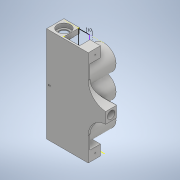
# Autodesk Inventor part: rearAxelHolder 10-29
Saved by Autodesk Inventor 2020 (Build 240168000, 168)
## iProperties
Created: 2019-10-24
Part Number: rearAxelHolder 10-29
Material: Generic
Document SubType Name: Modeling
Designer: Aditya Kendre
Density: 1 g/cm^3
Appearance: Default
Author: Aditya Kendre
## iProperties of the stored document rearAxelHolder 10-24_3DPrint.ipt
Created: 2019-10-24
Part Number: rearAxelHolder 10-24_3DPrint
Material: Generic
Document SubType Name: Modeling
Designer: Aditya Kendre
Density: 1 g/cm^3
Appearance: Default
Author: Aditya Kendre
Autodesk Inventor part; units mm, degrees
ref_plane "YZ Plane" through (0, 0, 0) normal (1, 0, 0) x (0, 1, 0)
ref_plane "XZ Plane" through (0, 0, 0) normal (0, 1, 0) x (-1, 0, 0)
ref_plane "XY Plane" through (0, 0, 0) normal (0, 0, 1) x (1, 0, 0)
sketch "Sketch1" plane through (0, 0, 0) normal (0, 1, 0) x (-1, 0, 0)
  line L0 (0, 0) -> (25, 0)
  line L1 (25, 0) -> (25, -165)
  line L2 (25, -165) -> (0, -165)
  line L3 (0, -165) -> (0, 0)
  dimension "d0" = 25
  dimension "d1" = 165
  constraints: 8 end point, 2 parallel, 1 horizontal, 1 perpendicular
  measures "d0" distance of L1.end L2.end
  measures "d1" distance of L0.end L1.end
extrude "Extrusion1" add sketch "Sketch1" along normal blind 3
sketch "Sketch2" plane through (0, 3, 0) normal (0, 1, 0) x (1, 0, 0)
  line L0 (0, 0) -> (0, 165) projected
  line L1 (-25, 165) -> (-25, 0) projected
  line L2 (0, 0) -> (-25, 0)
  line L3 (-25, 0) -> (-25, 8.5)
  line L4 (-25, 8.5) -> (0, 8.5)
  line L5 (0, 8.5) -> (0, 0)
  line L6 (-25, 165) -> (0, 165)
  line L7 (0, 165) -> (0, 156.5)
  line L8 (0, 156.5) -> (-25, 156.5)
  line L9 (-25, 156.5) -> (-25, 165)
  dimension "d4" = 8.5
  dimension "d5" = 8.5
  constraints: 16 end point, 4 parallel, 2 horizontal, 2 perpendicular, 2 point on line
  measures "d4" distance of L2.end L3.end
  measures "d5" distance of L6.end L7.end
extrude "Extrusion2" add sketch "Sketch2" along normal blind 25 contours L2 L1 L4 L0 | L8 L1 L6 L0
sketch "Sketch3" plane through (-25, 0, 0) normal (0, 0, 1) x (1, 0, 0)
  line L0 (0, 3) -> (0, 28) construction
  line L1 (25, 3) -> (25, 28) construction
  line L2 (0, 28) -> (25, 28) construction
  line L3 (25, 28) -> (25, 3) construction
  line L4 (25, 3) -> (0, 3) construction
  line L5 (0, 3) -> (0, 28) construction
  circle A0 centre (12.5, 15.5) radius 11.375
  point P0 (25, 0)
  dimension "d8" = 25
  dimension "d9" = 22.75
  constraints: 8 end point, 2 parallel, 1 centre point, 1 horizontal, 1 perpendicular
  measures "d8" distance of L2.end L1.start
  measures "d9" diameter of A0
extrude "Extrusion3" cut sketch "Sketch3" against normal blind 7.1
sketch "Sketch4" plane through (-25, 0, 0) normal (0, 0, 1) x (1, 0, 0)
  circle A0 centre (12.5, 15.5) radius 11.375 projected
  circle A1 centre (12.5, 15.5) radius 7.75
  point P0 (25, 0)
  dimension "d12" = 15.5
  constraints: 1 centre point, 1 coincident
  measures "d12" diameter of A1
extrude "Extrusion4" cut sketch "Sketch4" against normal blind 165 contours A1
sketch "Sketch5" plane through (0, 0, -165) normal (0, 0, -1) x (-1, 0, 0)
  circle A0 centre (12.5, 15.5) radius 7.75 projected
  circle A1 centre (12.5, 15.5) radius 11
  point P0 (0, 0)
  constraints: 1 centre point, 1 coincident
extrude "Extrusion5" cut sketch "Sketch5" against normal blind 7.1
sketch "Sketch6" plane through (0, 3, 0) normal (0, 1, 0) x (1, 0, 0)
  line L0 (-25, 156.5) -> (-25, 8.5) projected
  line L1 (-20.25, 8.5) -> (-4.75, 8.5) projected
  line L2 (-25, 156.5) -> (-20, 156.5)
  line L3 (-20, 156.5) -> (-20, 8.5)
  line L4 (-20, 8.5) -> (-25, 8.5)
  line L5 (-25, 8.5) -> (-25, 156.5)
  line L6 (0, 8.5) -> (0, 156.5) projected
  line L7 (-4.75, 156.5) -> (-20.25, 156.5) projected
  line L8 (0, 8.5) -> (-5, 8.5)
  line L9 (-5, 8.5) -> (-5, 156.5)
  line L10 (-5, 156.5) -> (0, 156.5)
  line L11 (0, 156.5) -> (0, 8.5)
  point P0 (0, 0)
  dimension "d17" = 5
  dimension "d18" = 5
  constraints: 16 end point, 4 parallel, 2 horizontal, 2 perpendicular, 2 point on line
  measures "d17" distance of L3.end L4.end
  measures "d18" distance of L9.end L10.end
extrude "Extrusion6" add sketch "Sketch6" along normal blind 10 contours L2 L3 L1 L4 L0 | L7 L10 L6 L8 L1 L9
fillet "Fillet1" radius 2 2 edges at (-5, 13, -82.5) (-20, 13, -82.5)
sketch "Sketch7" plane through (0, 0, 0) normal (1, 0, 0) x (0, 0, -1)
  line L0 (165, 0) -> (0, 0) projected
  line L1 (0, 0) -> (16, 0)
  line L2 (16, 0) -> (16, 8)
  line L3 (16, 8) -> (0, 8)
  line L4 (0, 8) -> (0, 0)
  line L5 (165, 0) -> (149, 0)
  line L6 (149, 0) -> (149, 8)
  line L7 (149, 8) -> (165, 8)
  line L8 (165, 8) -> (165, 0)
  line L9 (0, 28) -> (8.5, 28) projected
  line L10 (0, 28) -> (16, 28)
  line L11 (16, 28) -> (16, 20)
  line L12 (16, 20) -> (0, 20)
  line L13 (0, 20) -> (0, 28)
  line L14 (165, 0) -> (165, 28) projected
  line L15 (165, 28) -> (149, 28)
  line L16 (149, 28) -> (149, 20)
  line L17 (149, 20) -> (165, 20)
  line L18 (165, 20) -> (165, 28)
  dimension "d22" = 16
  dimension "d23" = 8
  dimension "d24" = 16
  dimension "d25" = 16
  dimension "d26" = 8
  constraints: 32 end point, 8 parallel, 4 horizontal, 4 perpendicular, 3 point on line
  measures "d22" distance of L3.end L2.end
  measures "d23" distance of L2.end L1.end
  measures "d24" distance of L6.end L7.end
  measures "d25" distance of L11.end L12.end
  measures "d26" distance of L10.end L11.end
extrude "Extrusion7" add sketch "Sketch7" along normal blind 45
fillet "Fillet2" radius 6 2 edges at (0, 24, -156.5) (0, 24, -8.5)
sketch "Sketch8" plane through (45, 0, 0) normal (1, 0, 0) x (0, 0, -1)
  line L0 (8.5, 20) -> (0, 20) construction
  line L1 (16, 28) -> (16, 20) construction
  line L2 (0, 20) -> (16, 28) construction
  line L3 (0, 0) -> (165, 0) construction
  line L4 (16, 8) -> (16, 0) construction
  line L5 (0, 0) -> (16, 8) construction
  line L6 (150.5, 28) -> (149, 28) construction
  line L7 (165, 8) -> (165, 20) construction
  line L8 (149, 28) -> (165, 20) construction
  line L9 (149, 0) -> (149, 8) construction
  line L10 (149, 8) -> (165, 0) construction
  line L11 (163.125, 22.25) -> (150.875, 22.25)
  line L12 (150.875, 22.25) -> (150.875, 25.75)
  line L13 (150.875, 25.75) -> (163.125, 25.75)
  line L14 (163.125, 25.75) -> (163.125, 22.25)
  line L15 (163.125, 22.25) -> (150.875, 25.75) construction
  line L16 (150.875, 22.25) -> (163.125, 25.75) construction
  line L17 (163.125, 2.25) -> (150.875, 2.25)
  line L18 (150.875, 2.25) -> (150.875, 5.75)
  line L19 (150.875, 5.75) -> (163.125, 5.75)
  line L20 (163.125, 5.75) -> (163.125, 2.25)
  line L21 (163.125, 2.25) -> (150.875, 5.75) construction
  line L22 (150.875, 2.25) -> (163.125, 5.75) construction
  line L23 (14.125, 22.25) -> (1.875, 22.25)
  line L24 (1.875, 22.25) -> (1.875, 25.75)
  line L25 (1.875, 25.75) -> (14.125, 25.75)
  line L26 (14.125, 25.75) -> (14.125, 22.25)
  line L27 (14.125, 22.25) -> (1.875, 25.75) construction
  line L28 (1.875, 22.25) -> (14.125, 25.75) construction
  line L29 (14.125, 2.25) -> (1.875, 2.25)
  line L30 (1.875, 2.25) -> (1.875, 5.75)
  line L31 (1.875, 5.75) -> (14.125, 5.75)
  line L32 (14.125, 5.75) -> (14.125, 2.25)
  line L33 (14.125, 2.25) -> (1.875, 5.75) construction
  line L34 (1.875, 2.25) -> (14.125, 5.75) construction
  point P0 (157, 24)
  point P1 (157, 4)
  point P2 (8, 24)
  point P3 (8, 4)
  dimension "d30" = 12.25
  dimension "d31" = 3.5
  dimension "d32" = 12.25
  dimension "d33" = 3.5
  dimension "d34" = 12.25
  dimension "d35" = 12.25
  dimension "d36" = 3.5
  constraints: 56 end point, 12 midpoint, 8 parallel, 4 horizontal, 4 perpendicular, 1 point on line
  measures "d30" distance of L12.end L13.end
  measures "d31" distance of L11.end L12.end
  measures "d32" distance of L18.end L19.end
  measures "d33" distance of L17.end L18.end
  measures "d34" distance of L24.end L25.end
  measures "d35" distance of L30.end L31.end
  measures "d36" distance of L29.end L30.end
extrude "Extrusion8" cut sketch "Sketch8" against normal blind 40
sketch "Sketch9" plane through (0, 8, 0) normal (0, 1, 0) x (1, 0, 0)
  line L0 (0, 0) -> (0, 16) construction
  line L1 (0, 8) -> (0, 9) construction
  line L2 (45, 1.875) -> (45, 14.125) construction
  line L3 (0, 9) -> (45, 9) construction
  line L4 (45, 9) -> (45, 7) construction
  line L5 (45, 7) -> (0, 7) construction
  line L6 (0, 7) -> (0, 9) construction
  line L7 (0, 9) -> (45, 9)
  line L8 (45, 9) -> (45, 7)
  line L9 (45, 7) -> (0, 7)
  line L10 (0, 7) -> (0, 9)
  line L11 (0, 149) -> (0, 165) construction
  line L12 (0, 149) -> (0, 157) construction
  line L13 (0, 157) -> (0, 158) construction
  line L14 (45, 165) -> (45, 149) projected
  line L15 (0, 158) -> (45, 158)
  line L16 (45, 158) -> (45, 156)
  line L17 (45, 156) -> (0, 156)
  line L18 (0, 156) -> (0, 158)
  dimension "d39" = 1
  dimension "d40" = 2
  dimension "d41" = 8
  dimension "d42" = 1
  dimension "d43" = 2
  constraints: 30 end point, 6 parallel, 4 point on line, 3 horizontal, 3 perpendicular, 1 midpoint, 1 vertical
  measures "d39" distance of L1.start L1.end
  measures "d40" distance of L3.end L4.end
  measures "d41" distance of L11.start L12.end
  measures "d42" distance of L12.end L13.end
  measures "d43" distance of L15.end L16.end
extrude "Extrusion9" add sketch "Sketch9" along normal blind 12
fillet "Fillet3" radius 6 2 edges at (0, 16.5, -156.5) (0, 16.5, -8.5)
sketch "Sketch10" plane through (-25, 0, -165) normal (0, 0, -1) x (-1, 0, 0)
  circle A0 centre (-12.5, 15.5) radius 11.375 projected
  circle A1 centre (-12.5, 15.5) radius 11.375
  point P0 (-25, 0)
  constraints: 1 centre point, 1 coincident
extrude "Extrusion10" cut sketch "Sketch10" against normal blind 7.1
sketch "Sketch11" plane through (0, 0, 0) normal (0, -1, 0) x (1, 0, 0)
  line L0 (0, -16) -> (45, -16) projected
  line L1 (0, -149) -> (0, -16) projected
  line L2 (45, -16) -> (0, -16)
  line L3 (0, -16) -> (0, -149)
  line L4 (0, -149) -> (45, -149)
  line L5 (45, -149) -> (45, -16)
  point P0 (0, 0)
  constraints: 8 end point, 2 parallel, 1 horizontal, 1 perpendicular
extrude "Extrusion11" add sketch "Sketch11" against normal blind 3
sketch "Sketch12" plane through (0, 3, 0) normal (0, 1, 0) x (1, 0, 0)
  point P0 (0, 0)
sketch "Sketch13" plane through (0, 3, 0) normal (0, 1, 0) x (1, 0, 0)
  point P0 (0, 0)
sketch "Sketch14" plane through (0, 3, 0) normal (0, 1, 0) x (1, 0, 0)
  line L0 (45, 16) -> (45, 0) construction
  line L1 (0, 149) -> (45, 149) construction
  line L2 (45, 16) -> (3, 16) construction
  line L3 (3, 16) -> (3, 149) construction
  line L4 (3, 149) -> (45, 149) construction
  line L5 (45, 149) -> (45, 16) construction
  line L6 (3, 16) -> (45, 149) construction
  circle A0 centre (24, 82.5) radius 21
  circle A1 centre (24, 82.5) radius 19.375
  line L7 (24, 82.5) -> (24, 124.5) construction
  circle A2 centre (24, 124.5) radius 21
  circle A3 centre (24, 124.5) radius 19.375
  line L8 (24, 82.5) -> (24, 40.5) construction
  circle A4 centre (24, 40.5) radius 21
  circle A5 centre (24, 40.5) radius 19.375
  point P0 (0, 0)
  dimension "d51" = 42
  dimension "d52" = 38.75
  dimension "d53" = 42
  dimension "d54" = 38.75
  dimension "d55" = 42
  dimension "d56" = 38.75
  constraints: 14 end point, 6 centre point, 5 coincident, 2 parallel, 2 tangent, 2 vertical, 1 horizontal, 1 midpoint, 1 perpendicular, 1 point on line
  measures "d51" distance of L3.end L4.end
  measures "d52" diameter of A1
  measures "d53" distance of L7.start L7.end
  measures "d54" diameter of A3
  measures "d55" distance of L7.start L8.end
  measures "d56" diameter of A5
extrude "Extrusion12" add sketch "Sketch14" along normal blind 45
sketch "Sketch15" plane through (24, 48, -40.5) normal (0, 1, 0) x (1, 0, 0)
  line L0 (0, 20.1158) -> (-2, 20.1158)
  line L1 (-2, 20.1158) -> (-2, 21.9714)
  line L2 (-2, 21.9714) -> (0, 21.9714)
  line L3 (0, 21.9714) -> (0, 20.1158)
  line L4 (-2, 21.9714) -> (2, 21.9714)
  line L5 (2, 21.9714) -> (2, 20.1158)
  line L6 (2, 20.1158) -> (-2, 20.1158)
  line L7 (-2, 20.1158) -> (-2, 21.9714)
  line L8 (0, 62.262) -> (-2, 62.262)
  line L9 (-2, 62.262) -> (-2, 63.8269)
  line L10 (-2, 63.8269) -> (0, 63.8269)
  line L11 (0, 63.8269) -> (0, 62.262)
  line L12 (-2, 63.8269) -> (2, 63.8269)
  line L13 (2, 63.8269) -> (2, 62.262)
  line L14 (2, 62.262) -> (-2, 62.262)
  line L15 (-2, 62.262) -> (-2, 63.8269)
  point P0 (-24, -40.5)
  dimension "d59" = 2
  dimension "d60" = 4
  dimension "d61" = 2
  dimension "d62" = 4
  constraints: 32 end point, 8 parallel, 4 horizontal, 4 perpendicular, 3 point on line
  measures "d59" distance of L1.end L2.end
  measures "d60" distance of L5.end L6.end
  measures "d61" distance of L9.end L10.end
  measures "d62" distance of L13.end L14.end
extrude "Extrusion13" add sketch "Sketch15" against normal blind 45
sketch "Sketch16" plane through (0, 28, 0) normal (0, 1, 0) x (1, 0, 0)
  circle A0 centre (24, 40.5) radius 19.375 construction
  line L0 (24, 40.5) -> (24, 0) construction
  line L1 (24, 0) -> (14, 0) construction
  line L2 (-25, 0) -> (45, 0) construction
  line L3 (0, 165) -> (45, 165) projected
  line L4 (19, 0) -> (0, 0)
  line L5 (0, 0) -> (0, 165)
  line L6 (0, 165) -> (19, 165)
  line L7 (19, 165) -> (19, 0)
  dimension "d65" = 10
  constraints: 12 end point, 2 parallel, 2 point on line, 1 horizontal, 1 perpendicular, 1 vertical
  measures "d65" distance of L0.end L1.end
sketch "Sketch17" plane through (0, 8, 0) normal (0, 1, 0) x (1, 0, 0)
  line L0 (0, 14.5) -> (0, 16) projected
  line L1 (-25, 0) -> (45, 0) projected
  line L2 (0, 16) -> (45, 16)
  line L3 (45, 16) -> (45, 0)
  line L4 (45, 0) -> (0, 0)
  line L5 (0, 0) -> (0, 16)
  line L6 (0, 165) -> (45, 165) projected
  line L7 (0, 149) -> (45, 149) projected
  line L8 (0, 165) -> (45, 165)
  line L9 (45, 165) -> (45, 149)
  line L10 (45, 149) -> (0, 149)
  line L11 (0, 149) -> (0, 165)
  constraints: 16 end point, 4 parallel, 2 horizontal, 2 perpendicular
extrude "Extrusion14" add sketch "Sketch17" along normal blind 12
sketch "Sketch18" plane through (-25, 0, -165) normal (-1, 0, 0) x (0, 0, 1)
  line L0 (0, 28) -> (16, 28) projected
  line L1 (156.5, 13) -> (8.5, 13) projected
  line L2 (0, 28) -> (8.5, 28)
  line L3 (8.5, 28) -> (8.5, 13)
  line L4 (8.5, 13) -> (0, 13)
  line L5 (0, 13) -> (0, 28)
  line L6 (156.5, 13) -> (156.5, 28) projected
  line L7 (165, 26.875) -> (165, 4.125) projected
  line L8 (156.5, 28) -> (165, 28)
  line L9 (165, 28) -> (165, 13)
  line L10 (165, 13) -> (156.5, 13)
  line L11 (156.5, 13) -> (156.5, 28)
  line L12 (165, 0) -> (0, 0)
  line L13 (0, 0) -> (0, 13)
  line L14 (0, 13) -> (165, 13)
  line L15 (165, 13) -> (165, 0)
  constraints: 24 end point, 6 parallel, 3 horizontal, 3 perpendicular, 2 point on line
extrude "Extrusion15" add sketch "Sketch18" along normal blind 2
sketch "Sketch19" plane through (0, 28, 0) normal (0, 1, 0) x (1, 0, 0)
  line L0 (45, 16) -> (45, 0) projected
  line L1 (0, 16) -> (0, 149) projected
  line L2 (45, 0) -> (0, 0)
  line L3 (0, 0) -> (0, 16)
  line L4 (0, 16) -> (45, 16)
  line L5 (45, 16) -> (45, 0)
  line L6 (-22, 8.5) -> (-27, 8.5) projected
  line L7 (0, 0) -> (-27, 0)
  line L8 (-27, 0) -> (-27, 8.5)
  line L9 (-27, 8.5) -> (0, 8.5)
  line L10 (0, 8.5) -> (0, 0)
  line L11 (0, 149) -> (45, 149) projected
  line L12 (-27, 165) -> (45, 165) projected
  line L13 (45, 149) -> (0, 149)
  line L14 (0, 149) -> (0, 165)
  line L15 (0, 165) -> (45, 165)
  line L16 (45, 165) -> (45, 149)
  line L17 (-27, 156.5) -> (-22, 156.5) projected
  line L18 (-27, 156.5) -> (0, 156.5)
  line L19 (0, 156.5) -> (0, 165)
  line L20 (0, 165) -> (-27, 165)
  line L21 (-27, 165) -> (-27, 156.5)
  arc A0 (0, 150.5) -> (-6, 156.5) centre (-6, 150.5) ccw projected
  arc A1 (0, 150.5) -> (-6, 156.5) centre (-6, 150.5) ccw
  arc A2 (-6, 8.5) -> (0, 14.5) centre (-6, 14.5) ccw projected
  arc A3 (-6, 8.5) -> (0, 14.5) centre (-6, 14.5) ccw
  constraints: 32 end point, 8 parallel, 5 point on circle, 4 horizontal, 4 perpendicular, 3 point on line, 2 centre point
extrude "Extrusion16" add sketch "Sketch19" along normal blind 2
sketch "Sketch20" plane through (-27, 0, -165) normal (-1, 0, 0) x (0, 0, 1)
  line L0 (83.5, 4) -> (81.5, 4)
  line L1 (81.5, 4) -> (81.5, 6)
  line L2 (81.5, 6) -> (83.5, 6)
  line L3 (83.5, 6) -> (83.5, 4)
  line L4 (83.5, 4) -> (81.5, 6) construction
  line L5 (81.5, 4) -> (83.5, 6) construction
  point P0 (165, 0)
  point P1 (82.5, 5000)
  point P2 (82.5, 5)
  dimension "d72" = 2
  dimension "d73" = 2
  constraints: 12 end point, 2 midpoint, 2 parallel, 1 horizontal, 1 perpendicular
  measures "d72" distance of L1.end L2.end
  measures "d73" distance of L0.end L1.end
extrude "Extrusion17" cut sketch "Sketch20" against normal blind 5
sketch "Sketch21" plane through (0, 0, 0) normal (0, -1, 0) x (1, 0, 0)
  line L0 (-21, -81.5) -> (-23, -81.5)
  line L1 (-23, -81.5) -> (-23, -83.5)
  line L2 (-23, -83.5) -> (-21, -83.5)
  line L3 (-21, -83.5) -> (-21, -81.5)
  line L4 (-21, -81.5) -> (-23, -83.5) construction
  line L5 (-23, -81.5) -> (-21, -83.5) construction
  point P0 (0, 0)
  point P1 (-22, -82.5)
  dimension "d76" = 2
  dimension "d77" = 2
  constraints: 12 end point, 2 midpoint, 2 parallel, 1 horizontal, 1 perpendicular
  measures "d76" distance of L2.end L1.end
  measures "d77" distance of L1.end L0.end
extrude "Extrusion18" cut sketch "Sketch21" against normal blind 7
fillet "Fillet4" radius 1 3 edges at (-27, 4, -82.5) (-23, 0, -82.5) (-23, 4, -82.5)
sketch "Sketch22" plane through (45, 0, 0) normal (1, 0, 0) x (0, 0, -1)
  line L0 (14.125, 22.25) -> (1.875, 22.25) projected
  line L1 (14.125, 25.75) -> (14.125, 22.25) projected
  line L2 (1.875, 22.25) -> (14.125, 22.25)
  line L3 (14.125, 22.25) -> (14.125, 22.5)
  line L4 (14.125, 22.5) -> (1.875, 22.5)
  line L5 (1.875, 22.5) -> (1.875, 22.25)
  line L6 (163.125, 22.25) -> (150.875, 22.25) projected
  line L7 (163.125, 25.75) -> (163.125, 22.25) projected
  line L8 (150.875, 22.25) -> (163.125, 22.25)
  line L9 (163.125, 22.25) -> (163.125, 22.5)
  line L10 (163.125, 22.5) -> (150.875, 22.5)
  line L11 (150.875, 22.5) -> (150.875, 22.25)
  point P0 (0, 0)
  dimension "d81" = 0.25
  dimension "d82" = 0.25
  constraints: 16 end point, 4 parallel, 2 horizontal, 2 perpendicular, 2 point on line
  measures "d81" distance of L3.end L2.end
  measures "d82" distance of L9.end L8.end
extrude "Extrusion19" add sketch "Sketch22" against normal blind 44.75
sketch "Sketch23" plane through (45, 0, 0) normal (1, 0, 0) x (0, 0, -1)
  line L0 (1.875, 5.75) -> (14.125, 5.75) projected
  line L1 (14.125, 5.75) -> (14.125, 2.25) projected
  line L2 (1.875, 5.75) -> (14.125, 5.75)
  line L3 (14.125, 5.75) -> (14.125, 2.25)
  line L4 (14.125, 2.25) -> (1.875, 2.25)
  line L5 (1.875, 2.25) -> (1.875, 5.75)
  line L6 (150.875, 5.75) -> (163.125, 5.75) projected
  line L7 (163.125, 2.25) -> (150.875, 2.25) projected
  line L8 (150.875, 5.75) -> (163.125, 5.75)
  line L9 (163.125, 5.75) -> (163.125, 2.25)
  line L10 (163.125, 2.25) -> (150.875, 2.25)
  line L11 (150.875, 2.25) -> (150.875, 5.75)
  point P0 (0, 0)
  constraints: 16 end point, 4 parallel, 2 horizontal, 2 perpendicular
extrude "Extrusion20" add sketch "Sketch23" against normal blind 44
sketch "Sketch24" plane through (-27, 0, 0) normal (0, 0, 1) x (1, 0, 0)
  circle A0 centre (14.5, 15.5) radius 11.375 projected
  circle A1 centre (14.5, 15.5) radius 11.375
  circle A2 centre (14.5, 15.5) radius 11.3
  point P0 (27, 0)
  dimension "d87" = 22.6
  constraints: 2 centre point, 2 coincident
  measures "d87" diameter of A2
extrude "Extrusion21" add sketch "Sketch24" against normal blind 8.5
sketch "Sketch25" plane through (45, 0, -165) normal (0, 0, -1) x (-1, 0, 0)
  circle A0 centre (57.5, 15.5) radius 11.375 projected
  circle A1 centre (57.5, 15.5) radius 11.375
  circle A2 centre (57.5, 15.5) radius 11.3
  point P0 (45, 0)
  dimension "d90" = 22.6
  constraints: 2 centre point, 2 coincident
  measures "d90" diameter of A2
extrude "Extrusion22" add sketch "Sketch25" against normal blind 8.5
sketch "Sketch26" plane through (0, 30, 0) normal (0, 1, 0) x (1, 0, 0)
  line L0 (45, 16) -> (45, 40.5) projected
  line L1 (0, 0) -> (45, 0)
  line L2 (45, 0) -> (45, 16)
  line L3 (45, 16) -> (0, 16)
  line L4 (0, 16) -> (0, 0)
  line L5 (0, 150.5) -> (0, 149) projected
  line L6 (-27, 165) -> (45, 165) projected
  line L7 (0, 149) -> (45, 149)
  line L8 (45, 149) -> (45, 165)
  line L9 (45, 165) -> (0, 165)
  line L10 (0, 165) -> (0, 149)
  constraints: 16 end point, 4 parallel, 2 horizontal, 2 perpendicular
extrude "Extrusion23" cut sketch "Sketch26" against normal blind 27
sketch "Sketch27" plane through (0, 0, 0) normal (0, -1, 0) x (1, 0, 0)
  line L0 (15, -92.025) -> (75, -92.025)
  line L1 (75, -92.025) -> (75, -72.975)
  line L2 (75, -72.975) -> (15, -72.975)
  line L3 (15, -72.975) -> (15, -92.025)
  line L4 (45, 0) -> (45, -165) projected
  line L5 (15, -92.025) -> (75, -72.975) construction
  line L6 (75, -92.025) -> (15, -72.975) construction
  point P0 (0, 0)
  point P1 (45, -82.5)
  point P2 (45, -72.975)
  point P3 (45, -92.025)
  dimension "d95" = 60
  dimension "d96" = 19.05
  constraints: 12 end point, 3 midpoint, 2 parallel, 1 horizontal, 1 perpendicular
  measures "d95" distance of L2.end L1.end
  measures "d96" distance of L1.end L0.end
extrude "Extrusion24" add sketch "Sketch27" against normal blind 3 contours L4 L2 L1 L0
fillet "Fillet5" radius 31.75 2 edges at (45, 1.5, -72.975) (45, 1.5, -92.025)
sketch "Sketch28" plane through (75, 0, -72.975) normal (1, 0, 0) x (0, 0, -1)
  line L0 (19.05, 0) -> (0, 0) projected
  line L1 (0, 0) -> (19.05, 0)
  line L2 (19.05, 0) -> (19.05, 19.05)
  line L3 (19.05, 19.05) -> (0, 19.05)
  line L4 (0, 19.05) -> (0, 0)
  point P0 (-72.975, 0)
  dimension "d100" = 19.05
  dimension "d101" = 19.05
  constraints: 8 end point, 2 parallel, 1 horizontal, 1 perpendicular
  measures "d100" distance of L3.end L2.end
  measures "d101" distance of L2.end L1.end
extrude "Extrusion25" add sketch "Sketch28" against normal blind 31.5
fillet "Fillet6" radius 38 2 edges at (59.25, 3, -92.025) (59.25, 3, -72.975)
sketch "Sketch29" plane through (75, 0, -72.975) normal (1, 0, 0) x (0, 0, -1)
  circle A0 centre (9.525, 9.525) radius 6.477
  point P0 (-72.975, 0)
  dimension "d105" = 12.954
  constraints: 1 centre point
  measures "d105" diameter of A0
extrude "Extrusion26" cut sketch "Sketch29" against normal blind 27.5
sketch "Sketch30" plane through (0, 3, 0) normal (0, 1, 0) x (1, 0, 0)
  line L0 (45, 0) -> (27, 0)
  line L1 (27, 0) -> (27, 18)
  line L2 (27, 18) -> (45, 18)
  line L3 (45, 18) -> (45, 0)
  line L4 (45, 123.7267) -> (45, 165) projected
  line L5 (45, 165) -> (27, 165)
  line L6 (27, 165) -> (27, 147)
  line L7 (27, 147) -> (45, 147)
  line L8 (45, 147) -> (45, 165)
  point P0 (0, 0)
  dimension "d108" = 18
  dimension "d109" = 18
  dimension "d110" = 18
  dimension "d111" = 18
  constraints: 16 end point, 4 parallel, 2 horizontal, 2 perpendicular
  measures "d108" distance of L1.end L2.end
  measures "d109" distance of L0.end L1.end
  measures "d110" distance of L7.end L6.end
  measures "d111" distance of L6.end L5.end
extrude "Extrusion27" add sketch "Sketch30" along normal blind 18
sketch "Sketch31" plane through (45, 0, 0) normal (1, 0, 0) x (0, 0, -1)
  line L0 (18, 3) -> (18, 21) construction
  line L1 (18, 21) -> (0, 21) construction
  line L2 (18, 3) -> (0, 21) construction
  circle A0 centre (9, 12) radius 1 construction
  circle A1 centre (9, 12) radius 1
  line L3 (147, 3) -> (147, 21) construction
  line L4 (147, 3) -> (165, 21) construction
  line L5 (165, 26.8) -> (165, 4.2) construction
  circle A2 centre (156, 12) radius 1
  point P0 (0, 0)
  dimension "d114" = 2
  dimension "d115" = 2
  dimension "d116" = 2
  constraints: 4 end point, 3 centre point, 2 coincident, 2 midpoint, 1 point on line
  measures "d114" diameter of A0
  measures "d115" diameter of A1
  measures "d116" diameter of A2
extrude "Extrusion28" cut sketch "Sketch31" against normal blind 5
sketch "Sketch32" plane through (-20, 3, -156.5) normal (0, 0, 1) x (1, 0, 0)
  line L0 (14, 27) -> (14, 17) projected
  line L1 (20, 27) -> (20, 0) projected
  line L2 (14, 27) -> (20, 27)
  line L3 (20, 27) -> (20, 17)
  line L4 (20, 17) -> (14, 17)
  line L5 (14, 17) -> (14, 27)
  point P0 (20, -3)
  dimension "d119" = 10
  constraints: 8 end point, 2 parallel, 1 horizontal, 1 perpendicular, 1 point on line
  measures "d119" distance of L2.end L3.end
extrude "Extrusion29" cut sketch "Sketch32" along normal blind 148
body "Solid1"
